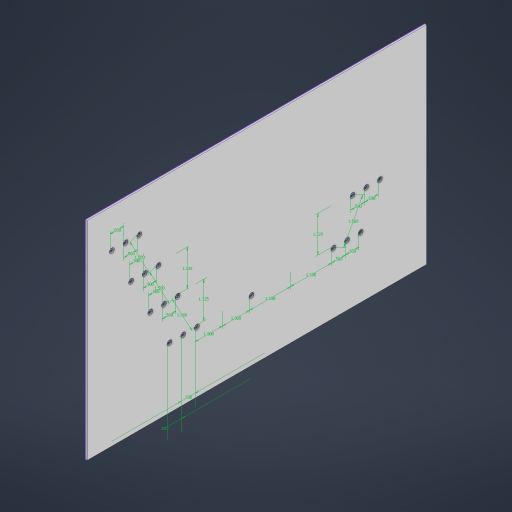
# Autodesk Inventor part: dtplate2
Saved by Autodesk Inventor 2024 (Build 280153000, 153)
## iProperties
Created: 2023-11-04
Part Number: dtplate2
Material: Generic
Document SubType Name: Modeling
Designer: macbook
Density: 1 g/cm^3
Appearance: Default
Author: macbook
Autodesk Inventor part; units mm, degrees
ref_plane "YZ Plane" through (0, 0, 0) normal (1, 0, 0) x (0, 1, 0)
ref_plane "XZ Plane" through (0, 0, 0) normal (0, 1, 0) x (-1, 0, 0)
ref_plane "XY Plane" through (0, 0, 0) normal (0, 0, 1) x (1, 0, 0)
sketch "Sketch1" plane through (0, 0, 0) normal (1, 0, 0) x (0, 1, 0)
  line L0 (0, 0) -> (0, 12.7)
  line L1 (0, 12.7) -> (0, 25.4)
  line L2 (0, 0) -> (33.655, 0)
  line L3 (0, 0) -> (33.655, 17.8592)
  line L4 (33.655, 17.8592) -> (67.31, 17.8592)
  line L5 (33.655, 17.8592) -> (67.31, 35.7184)
  line L6 (67.31, 35.7184) -> (100.965, 53.5776)
  line L7 (67.31, 35.7184) -> (100.965, 35.7184)
  line L8 (33.655, 17.8592) -> (33.655, 30.5592)
  line L9 (33.655, 30.5592) -> (33.655, 43.2592)
  line L10 (67.31, 35.7184) -> (67.31, 48.4184)
  line L11 (67.31, 48.4184) -> (67.31, 61.1184)
  line L12 (100.965, 53.5776) -> (100.965, 66.2776)
  line L13 (100.965, 66.2776) -> (100.965, 78.9776)
  line L14 (0, 0) -> (0, -25.4)
  line L15 (0, -25.4) -> (0, -50.8)
  line L16 (0, -50.8) -> (0, -88.9)
  line L17 (0, -88.9) -> (0, -127)
  line L18 (0, -127) -> (0, -139.7)
  line L19 (0, -139.7) -> (0, -152.4)
  line L20 (0, -127) -> (33.655, -127)
  line L21 (0, -127) -> (33.655, -144.8592)
  line L22 (33.655, -144.8592) -> (33.655, -157.5592)
  line L23 (33.655, -157.5592) -> (33.655, -170.2592)
  line L24 (136.7778, 101.8092) -> (-56.3816, 101.8092)
  line L25 (-56.3816, 101.8092) -> (-56.3816, -213.5728)
  line L26 (-56.3816, -213.5728) -> (136.7778, -213.5728)
  line L27 (136.7778, -213.5728) -> (136.7778, 101.8092)
  dimension "d78" = 12.7
  dimension "d79" = 12.7
  dimension "d81" = 33.655
  dimension "d82" = 38.1
  dimension "d83" = 33.655
  dimension "d84" = 38.1
  dimension "d85" = 38.1
  dimension "d86" = 12.7
  dimension "d87" = 12.7
  dimension "d88" = 12.7
  dimension "d89" = 12.7
  dimension "d90" = 12.7
  dimension "d91" = 12.7
  dimension "d92" = 25.4
  dimension "d93" = 25.4
  dimension "d94" = 38.1
  dimension "d95" = 38.1
  dimension "d96" = 12.7
  dimension "d97" = 12.7
  dimension "d98" = 33.655
  dimension "d99" = 38.1
  dimension "d100" = 12.7
  dimension "d101" = 12.7
  constraints: 56 end point, 19 coincident, 9 vertical, 8 point on line, 5 horizontal, 2 parallel, 1 perpendicular
  measures "d78" distance of L0.start L0.end
  measures "d79" distance of L0.end L1.end
  measures "d81" distance of L0.start L2.end
  measures "d82" distance of L0.start L3.end
  measures "d83" distance of L3.end L4.end
  measures "d84" distance of L3.end L5.end
  measures "d85" distance of L5.end L6.end
  measures "d86" distance of L3.end L8.end
  measures "d87" distance of L8.end L9.end
  measures "d88" distance of L5.end L10.end
  measures "d89" distance of L10.end L11.end
  measures "d90" distance of L6.end L12.end
  measures "d91" distance of L12.end L13.end
  measures "d92" distance of L0.start L14.end
  measures "d93" distance of L14.end L15.end
  measures "d94" distance of L15.end L16.end
  measures "d95" distance of L16.end L17.end
  measures "d96" distance of L17.end L18.end
  measures "d97" distance of L18.end L19.end
  measures "d98" distance of L20.start L20.end
  measures "d99" distance of L20.start L21.end
  measures "d100" distance of L22.start L22.end
  measures "d101" distance of L22.end L23.end
extrude "Extrusion1" add sketch "Sketch1" along normal blind 1.5875
hole "Hole4" at (0, 0, 0) at (0, 0, 12.7) at (0, 0, 25.4) at (0, 0, -127) at (0, 0, -139.7) at (0, 0, -152.4) at (0, 33.655, -144.8592) at (0, 0, -50.8) at (0, 100.965, 78.9776) at (0, 100.965, 66.2776) at (0, 100.965, 53.5776) at (0, 67.31, 61.1184) at (0, 67.31, 48.4184) at (0, 67.31, 35.7184) at (0, 33.655, 43.2592) at (0, 33.655, 30.5592) at (0, 33.655, 17.8592) at (0, 33.655, -157.5592) at (0, 33.655, -170.2592) direction (1, 0, 0) diameter 4.7625 end through all
body "Solid1"
